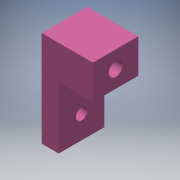
# Autodesk Inventor part: Hinge Block 2
Saved by Autodesk Inventor 2017 (Build 210142000, 142)
## iProperties
Created: 2017-01-24
Part Number: Hinge Block 2
Material: Generic
Document SubType Name: Modeling
Designer: Ben
Density: 1 g/cm^3
Appearance: Pink
Author: Ben
Autodesk Inventor part; units mm, degrees
ref_plane "YZ Plane" through (0, 0, 0) normal (1, 0, 0) x (0, 1, 0)
ref_plane "XZ Plane" through (0, 0, 0) normal (0, 1, 0) x (-1, 0, 0)
ref_plane "XY Plane" through (0, 0, 0) normal (0, 0, 1) x (1, 0, 0)
sketch "Sketch1" plane through (0, 0, 0) normal (1, 0, 0) x (0, 1, 0)
  line L0 (53.467, 12.7) -> (0, 12.7)
  line L1 (0, 12.7) -> (0, -12.7)
  line L2 (0, -12.7) -> (53.467, -12.7)
  line L3 (53.467, -12.7) -> (53.467, 12.7)
  line L4 (0, 0) -> (43.942, 0) construction
  circle A0 centre (43.942, 0) radius 3.81
  circle A1 centre (43.942, 0) radius 4.7625 construction
  circle A2 centre (28.575, 0) radius 3.175
  circle A3 centre (12.7, 0) radius 3.175
  dimension "d0" = 43.942
  dimension "d1" = 25.4
  dimension "d2" = 9.525
  dimension "d3" = 7.62
  dimension "d4" = 9.525
  dimension "d5" = 6.35
  dimension "d6" = 6.35
  dimension "d7" = 12.7
  dimension "d8" = 15.875
  constraints: 10 end point, 4 centre point, 3 coincident, 2 horizontal, 2 parallel, 2 point on line, 1 midpoint, 1 perpendicular
  measures "d0" distance of L4.start L4.end
  measures "d1" distance of L2.end L0.start
  measures "d2" distance from line of L4.end L3
  measures "d3" diameter of A0
  measures "d4" diameter of A1
  measures "d5" diameter of A2
  measures "d6" diameter of A3
  measures "d7" distance from line of L1 A3.centre
  measures "d8" distance of A3.centre A2.centre
extrude "Extrusion1" add sketch "Sketch1" along normal blind 28.575
sketch "Sketch2" plane through (0, 0, 12.7) normal (0, 0, 1) x (1, 0, 0)
  line L0 (0, 0) -> (28.575, 0) construction
  line L1 (28.575, 0) -> (9.525, 0)
  line L2 (9.525, 0) -> (9.525, 34.417)
  line L3 (9.525, 34.417) -> (28.575, 34.417)
  line L4 (28.575, 34.417) -> (28.575, 0)
  line L5 (0, 53.467) -> (28.575, 53.467) construction
  line L6 (0, 53.467) -> (0, 0) construction
  dimension "d12" = 19.05
  dimension "d14" = 9.525
  constraints: 8 end point, 2 parallel, 1 horizontal, 1 perpendicular
  measures "d12" distance between parallel lines of L5 L3
  measures "d14" distance between parallel lines of L6 L2
extrude "Extrusion2" cut sketch "Sketch2" against normal through all
body "Solid1"
